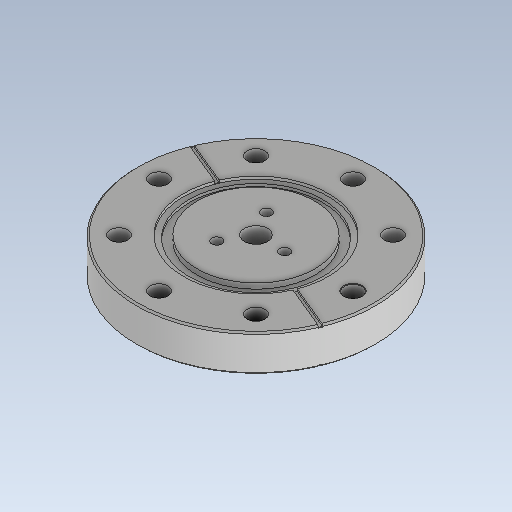
# Autodesk Inventor part: 4.5 flange
Saved by Autodesk Inventor 2020 (Build 240168000, 168)
## iProperties
Created: 2019-06-19
Part Number: 4.5 flange
Material: Generic
Document SubType Name: Modeling
Designer: ColinP
Density: 1 g/cm^3
Appearance: Default
Mass: 159.214 g
Surface Area: 320.601 cm^2
Volume: 159.214 cm^3
Author: ColinP
Autodesk Inventor part; units mm, degrees
ref_plane "YZ Plane" through (0, 0, 0) normal (1, 0, 0) x (0, 1, 0)
ref_plane "XZ Plane" through (0, 0, 0) normal (0, 1, 0) x (-1, 0, 0)
ref_plane "XY Plane" through (0, 0, 0) normal (0, 0, 1) x (1, 0, 0)
sketch "Sketch1" plane through (0, 0, 0) normal (0, 1, 0) x (-1, 0, 0)
  circle A0 centre (0, 0) radius 56.769
  circle A1 centre (0, 0) radius 46.0756
  circle A2 centre (0, 0) radius 31.75
  dimension "d0" = 113.538
  dimension "d1" = 92.1512
  dimension "d2" = 63.5
  constraints: 3 centre point, 3 coincident
  measures "d0" diameter of A0
  measures "d1" diameter of A1
  measures "d2" diameter of A2
extrude "Extrusion1" add sketch "Sketch1" along normal blind 17.272 contours A0 | A1 | A2
sketch "Sketch2" plane through (0, 17.272, 0) normal (0, 1, 0) x (1, 0, 0)
  circle A0 centre (0, 0) radius 46.0756
  circle A1 centre (-46.0756, 0) radius 4.0894
  dimension "d5" = 92.1512
  dimension "d6" = 8.1788
  constraints: 1 centre point, 1 coincident, 1 horizontal alignment, 2 other
  measures "d6" diameter of A1
hole "Hole1" at (-46.0756, 17.272, 0) direction (0, -1, 0) diameter 8.4328 end through all
pattern_circular "Circular Pattern1" count 8 over 360 about axis through (0, 0, 0) along (0, 1, 0) of "Hole1"
sketch "Sketch4" plane through (0, 17.272, 0) normal (0, 1, 0) x (1, 0, 0)
  circle A0 centre (0, 0) radius 14.7993
  constraints: 1 centre point, 1 coincident
hole "Hole2" at (0, 17.272, 0) direction (0, -1, 0) diameter 63.5 end through all
sketch "Sketch6" plane through (0, 0, 0) normal (0, 1, 0) x (-1, 0, 0)
  circle A0 centre (0, 0) radius 31.75
  circle A1 centre (0, 0) radius 19.05
  constraints: 2 centre point, 2 coincident
extrude "Extrusion3" add sketch "Sketch6" along normal blind 17.272
sketch "Sketch7" plane through (0, 17.272, 0) normal (0, 1, 0) x (1, 0, 0)
  circle A0 centre (0, 0) radius 34.29
  circle A1 centre (0, 0) radius 31.75
  circle A2 centre (0, 0) radius 25.4
  circle A3 centre (0, 0) radius 27.94
  dimension "d35" = 68.58
  dimension "d36" = 63.5
  dimension "d37" = 50.8
  dimension "d38" = 55.88
  constraints: 4 centre point, 4 coincident
  measures "d35" diameter of A0
  measures "d36" diameter of A1
  measures "d37" diameter of A2
  measures "d38" diameter of A3
extrude "Extrusion4" cut sketch "Sketch7" against normal blind 1.27 contours A0
sketch "Sketch9" plane through (0, 17.272, 0) normal (0, 1, 0) x (1, 0, 0)
  circle A0 centre (0, 0) radius 27.94
  circle A1 centre (0, 0) radius 31.75
  dimension "d45" = 55.88
  dimension "d46" = 63.5
  constraints: 2 centre point, 2 coincident
  measures "d45" diameter of A0
  measures "d46" diameter of A1
extrude "Extrusion6" cut sketch "Sketch9" against normal blind 2.54
chamfer "Chamfer1" distance 0.254 angle 45 1 edges at (-46.0756, 17.272, -4.2164)
chamfer "Chamfer2" distance 0.254 angle 45 1 edges at (-46.0756, 0, -4.2164)
chamfer "Chamfer3" distance 0.762 angle 45 2 edges at (56.769, 17.272, 0) (56.769, 0, 0)
sketch "Sketch10" plane through (0, 17.272, 0) normal (0, 1, 0) x (1, 0, 0)
  circle A0 centre (32.5804, 32.5804) radius 4.2164 projected
  circle A1 centre (46.0756, 0) radius 4.2164 projected
  line L0 (32.5804, 32.5804) -> (46.0756, 0)
  line L1 (46.0756, 0) -> (39.328, 16.2902)
  circle A2 centre (-46.0756, 0) radius 4.4704 projected
  circle A3 centre (-32.5804, -32.5804) radius 4.2164 projected
  line L2 (-46.0756, 0) -> (-32.5804, -32.5804)
  line L3 (39.328, 16.2902) -> (-39.328, -16.2902)
  line L4 (-39.328, -16.2902) -> (52.9444, 21.9303)
  line L5 (-39.328, -16.2902) -> (60.5469, -16.2902) construction
  line L6 (52.9444, 21.9303) -> (-52.9809, -21.9454)
  line L7 (39.328, 16.2902) -> (39.6342, 15.551)
  line L8 (39.6342, 15.551) -> (39.0218, 17.0294)
  line L9 (39.0218, 17.0294) -> (52.0886, 22.4418)
  line L10 (39.0218, 17.0294) -> (53.1652, 17.0294) construction
  line L11 (52.0886, 22.4418) -> (31.2876, 13.8258)
  line L12 (39.6342, 15.551) -> (52.7487, 20.9832)
  circle A4 centre (0, 0) radius 56.769 projected
  line L13 (39.6342, 15.551) -> (53.8292, 15.551) construction
  line L14 (52.7487, 20.9832) -> (52.7487, 20.9832)
  line L15 (52.7487, 20.9832) -> (31.9774, 12.3794)
  circle A5 centre (0, 0) radius 34.29 projected
  line L16 (31.2876, 13.8258) -> (52.0886, 22.4418)
  line L17 (52.0886, 22.4418) -> (52.7487, 20.9832)
  line L18 (52.0886, 22.4418) -> (31.2876, 13.8258)
  point P0 (31.365, 13.8578)
  dimension "d58" = 22.5
  dimension "d59" = 0.8001
  dimension "d60" = 1.6002
  dimension "d61" = 22.5
  dimension "d62" = 22.5
  constraints: 38 end point, 6 point on line, 3 equal length, 3 horizontal, 2 midpoint, 1 collinear, 1 parallel, 4 other
  measures "d58" angle of L5 L4
  measures "d59" distance of L1.end L7.end
  measures "d60" distance of L7.end L8.end
  measures "d61" angle of L10 L9
  measures "d62" angle of L13 L12
extrude "Extrusion7" cut sketch "Sketch10" against normal blind 1.016 contours L9 L17 L4 L0 | L0 L3 A5 L11 | L4 L17 L12 L0 | L0 L15 A5 L3
sketch "Sketch11" plane through (0, 17.272, 0) normal (0, 1, 0) x (1, 0, 0)
  line L0 (31.365, 13.8578) -> (51.4323, 22.17) projected
  line L1 (52.0446, 20.6916) -> (31.9774, 12.3794) projected
  line L2 (51.4323, 22.17) -> (31.365, 13.8578)
  line L3 (31.365, 13.8578) -> (-52.6609, -20.9468)
  line L4 (52.0446, 20.6916) -> (31.9774, 12.3794)
  circle A0 centre (0, 0) radius 56.769 projected
  line L5 (-52.1363, -22.4616) -> (31.9774, 12.3794)
  line L6 (-52.1363, -22.4616) -> (-52.6609, -20.9468)
  arc A1 (31.365, 13.8578) -> (31.9774, 12.3794) centre (0, 0) ccw projected
  circle A2 centre (0, 0) radius 34.29 projected
  line L7 (-31.365, -13.8578) -> (-31.9774, -12.3794)
  point P0 (-31.365, -13.8578)
  constraints: 12 end point, 4 point on line, 2 point on circle, 1 collinear, 2 other
extrude "Extrusion8" cut sketch "Sketch11" against normal blind 1.016 contours A1 L5 L6 L3
sketch "Sketch13" plane through (0, 0, 0) normal (0, -1, 0) x (1, 0, 0)
  circle A0 centre (0, 0) radius 27.94
  circle A1 centre (0, 0) radius 31.75
  circle A2 centre (0, 0) radius 34.29
  constraints: 3 centre point, 3 coincident
extrude "Extrusion9" cut sketch "Sketch13" against normal blind 2.54 contours A1
extrude "Extrusion10" cut sketch "Sketch13" against normal blind 1.27 contours A2
sketch "Sketch14" plane through (0, 0, 0) normal (0, -1, 0) x (1, 0, 0)
  line L0 (31.365, -13.8578) -> (52.0886, -22.4418) projected
  line L1 (52.7487, -20.9832) -> (31.9774, -12.3794) projected
  line L2 (-52.6609, 20.9468) -> (-31.9774, 12.3794) projected
  line L3 (-31.365, 13.8578) -> (-52.1363, 22.4616) projected
  line L4 (51.4323, -22.17) -> (52.0886, -22.4418) projected
  line L5 (52.0886, -22.4418) -> (31.365, -13.8578)
  arc A0 (52.7487, -20.9832) -> (-52.1363, 22.4616) centre (0, 0) ccw projected
  line L6 (31.9774, -12.3794) -> (52.7487, -20.9832)
  line L7 (52.7487, -20.9832) -> (52.0886, -22.4418)
  circle A1 centre (0, 0) radius 34.29 projected
  line L8 (-31.9774, 12.3794) -> (-31.365, 13.8578)
  circle A2 centre (0, 0) radius 56.769 projected
  line L9 (-52.1363, 22.4616) -> (-52.6609, 20.9468)
  constraints: 10 end point, 1 collinear, 1 parallel
extrude "Extrusion11" cut sketch "Sketch14" against normal blind 1.016 contours A1 L1 L7 L0
extrude "Extrusion12" cut sketch "Sketch14" against normal blind 1.016 contours L2 L9 L3 A1
sketch "Sketch15" plane through (0, 0, 0) normal (0, 1, 0) x (-1, 0, 0)
  circle A0 centre (0, 0) radius 19.05
  constraints: 1 centre point, 1 coincident
extrude "Extrusion13" add sketch "Sketch15" along normal blind 17.272
sketch "Sketch17" plane through (0, 0, 0) normal (0, -1, 0) x (1, 0, 0)
  circle A0 centre (0, 0) radius 27.94 projected
  constraints: 1 coincident
hole "Hole4" at (0, 0, 0) direction (0, 1, 0) diameter 10.9982 end through all
sketch "Sketch18" plane through (0, 0, 0) normal (0, -1, 0) x (1, 0, 0)
  line L0 (0, 0) -> (-13.6144, 0)
  dimension "d103" = 13.6144
  constraints: 2 end point, 1 horizontal
  measures "d103" distance of L0.start L0.end
hole "Hole5" at (-13.6144, 0, 0) direction (0, 1, 0) diameter 4.9022 end through all
pattern_circular "Circular Pattern5" count 3 over 360 about axis through (0, 161.4933, 0) along (0, -1, 0) of "Hole5"
body "Solid1"
